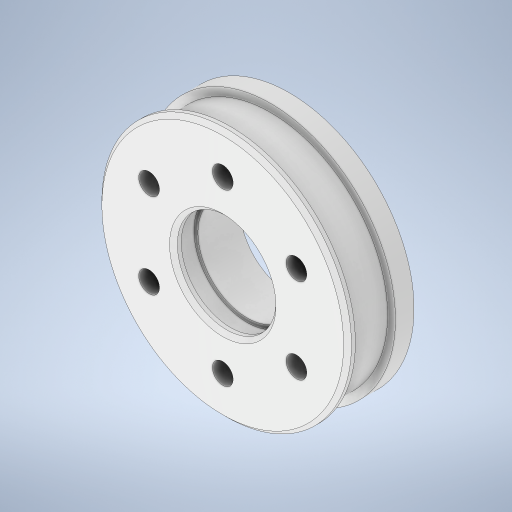
# Autodesk Inventor part: Spool Holder BAse
Saved by Autodesk Inventor 2024 (Build 280153000, 153)
## iProperties
Created: 2024-08-16
Part Number: Spool Holder BAse
Material: ABS Plastic
Document SubType Name: Modeling
Designer: Ishaan
Density: 1.06 g/cm^3
Appearance: Smooth - White
Author: Ishaan
Autodesk Inventor part; units mm, degrees
sketch "Sketch1" plane through (0, 0, 0) normal (0, 0, 1) x (1, 0, 0)
  circle A0 centre (0, 0) radius 29.9
  circle A1 centre (0, 0) radius 13.6
  dimension "d0" = 59.8
  dimension "d1" = 27.2
  constraints: 2 centre point, 2 coincident
  measures "d0" diameter of A0
  measures "d1" diameter of A1
extrude "Extrusion1" add sketch "Sketch1" against normal blind 15
ref_plane "Work Plane1" through (0, 0, -4.25) normal (0, 0, 1) x (1, 0, 0)
ref_plane "Work Plane2" through (0, 0, -10.25) normal (0, 0, 1) x (1, 0, 0)
sketch "Sketch2" plane through (0, 0, 0) normal (0, 0, 1) x (1, 0, 0)
  circle A0 centre (0, 0) radius 29.9 projected
  circle A1 centre (0, 0) radius 13.6 projected
  circle A2 centre (0, 0) radius 12.6
  circle A3 centre (0, 0) radius 31.9
  dimension "d4" = 1
  dimension "d8" = 2
  constraints: 2 centre point
  measures "d4" radial gap between concentric circles of A1 A2
  measures "d8" radial gap between concentric circles of A0 A3
extrude "Extrusion2" add sketch "Sketch2" against normal up to surface (10.75 mm away) from surface at -4.25 contours A1
extrude "Extrusion3" add sketch "Sketch2" against normal up to surface (4.75 mm away) from surface at -10.25 contours A3
sketch "Sketch8" plane through (0, 0, 0) normal (0, 0, 1) x (1, 0, 0)
  circle A0 centre (0, 0) radius 29.9 projected
  circle A1 centre (0, 0) radius 13.6 projected
  circle A2 centre (0, 0) radius 31.9 projected
  circle A3 centre (0, 0) radius 12.6 projected
extrude "Extrusion8" add sketch "Sketch8" along normal blind 2 contours A0 | A1 | A2
sketch "Sketch9" plane through (0, 0, 2) normal (0, 0, 1) x (1, 0, 0)
  circle A0 centre (0, 0) radius 29.9 projected
  circle A1 centre (0, 0) radius 29.9 projected
  circle A2 centre (0, 0) radius 13.6 projected
  circle A3 centre (0, 0) radius 13.6 projected
  line L0 (0, 29.9) -> (0, 13.6) construction
  point P0 (0, 21.75)
  constraints: 2 end point, 2 vertical alignment, 1 midpoint, 1 point on line, 1 vertical, 2 other
hole "Hole3" at (0, 21.75, 2) direction (0, 0, -1) diameter 5.3 end through all
pattern_circular "Circular Pattern2" count 6 over 360 about axis through (0, 0, 0) along (0, 0, 1) of "Hole3"
chamfer "Chamfer1" distance 1 angle 45 2 edges at (-31.9, 0, 2) (-12.6, 0, 2)
ref_plane "Work Plane5" through (0, 0, -5.125) normal (0, 0, -1) x (-1, 0, 0)
body "Solid1"
body "Solid4"
body "Solid5"
